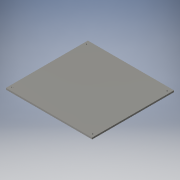
# Autodesk Inventor part: CustomBasePlate
Saved by Autodesk Inventor 2016 (Build 200138000, 138)
## iProperties
Created: 2015-08-31
Part Number: CustomBasePlate
Material: Aluminum 6061
Document SubType Name: Modeling
Designer: Tim
Density: 2.7 g/cm^3
Appearance: Aluminum - Flat
Author: Tim
Autodesk Inventor part; units mm, degrees
ref_plane "YZ Plane" through (0, 0, 0) normal (1, 0, 0) x (0, 1, 0)
ref_plane "XZ Plane" through (0, 0, 0) normal (0, 1, 0) x (-1, 0, 0)
ref_plane "XY Plane" through (0, 0, 0) normal (0, 0, 1) x (1, 0, 0)
sketch "Sketch1" plane through (0, 0, 0) normal (0, 1, 0) x (-1, 0, 0)
  line L0 (90.125, -106.756) -> (-131.875, -106.756)
  line L1 (-131.875, -106.756) -> (-131.875, 104.244)
  line L2 (-131.875, 104.244) -> (90.125, 104.244)
  line L3 (90.125, 104.244) -> (90.125, -106.756)
  line L4 (83.125, 94.744) -> (-124.875, -97.256) construction
  line L5 (-124.875, 94.744) -> (83.125, -97.256) construction
  circle A0 centre (83.125, -97.256) radius 2
  circle A1 centre (-124.875, -97.256) radius 2
  circle A2 centre (-124.875, 94.744) radius 2
  circle A3 centre (83.125, 94.744) radius 2
  point P0 (0, 0)
  point P1 (-20.875, -106.756)
  point P2 (90.125, -1.256)
  point P3 (-20.8729, -81.6668)
  point P4 (-124.8729, -81.6668)
  point P5 (-20.875, -1.256)
  dimension "d0" = 211
  dimension "d1" = 222
  dimension "d5" = 208
  dimension "d6" = 192
  dimension "d7" = 4
  dimension "d8" = 4
  dimension "d9" = 4
  dimension "d10" = 4
  constraints: 12 end point, 4 centre point, 4 coincident, 4 midpoint, 2 parallel, 1 horizontal, 1 perpendicular
  measures "d0" distance of L0.end L1.end
  measures "d1" distance of L1.end L2.end
  measures "d5" distance of L5.end L4.end
  measures "d6" distance of L5.end L4.start
  measures "d7" diameter of A0
  measures "d8" diameter of A1
  measures "d9" diameter of A2
  measures "d10" diameter of A3
extrude "Extrusion1" add sketch "Sketch1" along normal blind 4
body "Solid1"
